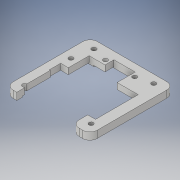
# Autodesk Inventor part: back-cam
Saved by Autodesk Inventor 2019 (Build 230136000, 136)
## iProperties
Created: 2019-02-22
Part Number: back-cam
Material: Generic
Document SubType Name: Modeling
Designer: Tesler
Density: 1 g/cm^3
Appearance: Default
Author: Tesler
Autodesk Inventor part; units mm, degrees
ref_plane "YZ Plane" through (0, 0, 0) normal (1, 0, 0) x (0, 1, 0)
ref_plane "XZ Plane" through (0, 0, 0) normal (0, 1, 0) x (-1, 0, 0)
ref_plane "XY Plane" through (0, 0, 0) normal (0, 0, 1) x (1, 0, 0)
sketch "Sketch1" plane through (0, 0, 0) normal (0, 1, 0) x (-1, 0, 0)
  line L0 (-29.924, 14.3694) -> (-29.924, -45.6306)
  line L1 (29.924, 14.3694) -> (29.924, -45.6306)
  line L2 (-7.574, -27.3788) -> (-7.574, -40.26)
  line L3 (-7.574, -40.26) -> (7.574, -40.26)
  line L4 (29.924, -45.6306) -> (-29.924, -45.6306)
  circle A0 centre (-23.749, 7.365) radius 1.5494
  arc A1 (23.749, 5.8156) -> (23.749, 8.9144) centre (23.749, 7.365) ccw
  circle A2 centre (10.414, -37.085) radius 1.5494
  line L5 (7.574, -33.91) -> (7.574, -40.26)
  circle A3 centre (23.6982, -25.782) radius 1.5494
  line L6 (7.574, -33.91) -> (18.924, -33.91)
  line L7 (-17.105, 14.3694) -> (-17.105, 3.065)
  line L8 (-22.624, 3.065) -> (-17.105, 3.065)
  line L9 (-22.624, 3.065) -> (-22.624, -27.3788)
  line L10 (-7.574, -27.3788) -> (-22.624, -27.3788)
  line L11 (18.924, -19.105) -> (18.924, -33.91)
  line L12 (18.924, -19.105) -> (24.424, -19.105)
  line L13 (23.749, -11.06) -> (24.424, -11.06)
  line L14 (24.424, -19.105) -> (24.424, -11.06)
  line L15 (-29.924, 14.3694) -> (-17.105, 14.3694)
  line L16 (22.1742, 14.3694) -> (29.924, 14.3694)
  line L17 (23.749, 5.8156) -> (23.7568, 5.8156)
  line L18 (23.749, 5.587) -> (23.749, -11.06)
  line L19 (22.1742, 14.3694) -> (22.1742, 8.9144)
  circle A4 centre (-10.414, -37.085) radius 1.5494
  line L20 (23.749, 5.587) -> (23.749, 5.8156)
  line L21 (23.749, 8.9144) -> (22.1742, 8.9144)
  point P0 (0, 0)
  point P1 (0, 0)
  dimension "d0" = 60
  dimension "d7" = 6.2258
  dimension "d8" = 19.8486
  dimension "d9" = 3.0988
  dimension "d12" = 12.8811
  dimension "d14" = 6.175
  dimension "d16" = 12.819
  dimension "d19" = 11
  dimension "d21" = 26.5256
  dimension "d22" = 34.5706
  dimension "d25" = 48.6956
  dimension "d27" = 5.5
  dimension "d28" = 6.175
  dimension "d30" = 7.3
  dimension "d31" = 11.7206
  dimension "d34" = 3.0988
  dimension "d35" = 3.0988
  dimension "d36" = 3.0988
  dimension "d38" = 8.5456
  dimension "d39" = 19.51
  dimension "d40" = 3.0988
  dimension "d41" = 8.5456
  dimension "d42" = 19.51
  dimension "d43" = 52.9956
  dimension "d44" = 6.175
  dimension "d176" = 5.455
  dimension "d177" = 7.7498
  constraints: 44 end point, 13 vertical, 10 horizontal, 5 centre point, 3 perpendicular, 2 point on circle, 1 coincident, 1 parallel, 1 point on line, 1 tangent
  measures "d0" distance of L0.start L0.end
  measures "d7" distance from line of L1 point (23.698, -25.782)
  measures "d8" distance from line of point (23.698, -25.782) L4
  measures "d9" diameter of A3
  measures "d12" distance of L2.start L2.end
  measures "d14" distance from line of A0.centre L0
  measures "d16" distance between parallel lines of L7 L0
  measures "d19" distance between parallel lines of L1 L11
  measures "d21" distance between parallel lines of L4 L12
  measures "d22" distance between parallel lines of L4 L13
  measures "d25" distance between parallel lines of L4 L8
  measures "d27" distance between parallel lines of L14 L1
  measures "d28" distance between parallel lines of L18 L1
  measures "d30" distance between parallel lines of L9 L0
  measures "d31" distance between parallel lines of L4 L6
  measures "d34" diameter of A1
  measures "d35" diameter of A0
  measures "d36" diameter of A2
  measures "d38" distance from line of L4 A2.centre
  measures "d39" distance from line of L1 A2.centre
  measures "d40" diameter of A4
  measures "d41" distance from line of L4 A4.centre
  measures "d42" distance from line of L0 A4.centre
  measures "d43" distance from line of L4 A0.centre
  measures "d44" distance from line of L1 A1.centre
  measures "d176" distance of L16.start L19.end
  measures "d177" distance between parallel lines of L1 L19
extrude "Extrusion1" add sketch "Sketch1" along normal blind 5.08 contours L15 L7 L8 L9 L10 L2 L3 L5 L6 L11 L12 L14 L13 L18 L20 A1 L21 L19 L16 L1 L4 L0 | A0 | A2 | A3 | A4
sketch "Sketch2" plane through (0, 0, 0) normal (0, -1, 0) x (1, 0, 0)
  line L0 (7.574, -40.26) -> (-7.574, -40.26) projected
  line L1 (-29.924, 14.3694) -> (-29.924, -45.6306) projected
  line L2 (-22.1742, 14.3694) -> (-29.924, 14.3694) projected
  line L3 (29.924, 14.3694) -> (17.105, 14.3694) projected
  line L4 (29.924, -45.6306) -> (29.924, 14.3694) projected
  line L5 (-26.924, 10.54) -> (26.924, 10.54)
  line L6 (-26.924, 10.54) -> (-26.924, -40.26)
  line L7 (-26.924, -40.26) -> (26.924, -40.26)
  line L8 (26.924, -40.26) -> (26.924, 10.54)
  point P0 (0, 0)
  dimension "d52" = 53.848
  dimension "d53" = 50.8
  constraints: 8 end point, 2 horizontal, 2 vertical, 1 parallel, 1 perpendicular
  measures "d52" distance of L5.start L5.end
  measures "d53" distance of L7.end L5.end
extrude "Extrusion3" cut sketch "Sketch2" against normal blind 0.7937
extrude "Extrusion2" cut sketch "Sketch1" along normal up to next contours A0 | A2 | A3 | A4
fillet "Fillet1" radius 5.08 4 edges at (29.924, 2.54, 14.3694) (29.924, 2.54, -45.6306) (-29.924, 2.54, -45.6306) (-29.924, 2.54, 14.3694)
fillet "Fillet2" radius 5.08 1 edges at (17.105, 2.54, 14.3694)
sketch "Sketch3" plane through (0, 0.7938, 0) normal (0, -1, 0) x (1, 0, 0)
  line L0 (-26.924, -40.26) -> (-26.924, 10.54) projected
  line L1 (-18.924, -33.91) -> (-7.574, -33.91) projected
  line L2 (-26.924, -40.26) -> (-14.224, -40.26)
  line L3 (-15.7226, -33.91) -> (-26.924, -33.91)
  line L4 (-26.924, -33.91) -> (-26.924, -40.26)
  line L5 (26.924, -40.26) -> (7.574, -40.26) projected
  line L6 (26.924, -40.26) -> (14.224, -40.26)
  line L7 (15.7226, -33.91) -> (26.924, -33.91)
  line L8 (26.924, -33.91) -> (26.924, -40.26)
  line L9 (-14.224, -40.26) -> (-14.224, -35.4086)
  line L10 (14.224, -40.26) -> (14.224, -35.4086)
  line L11 (14.224, -35.4086) -> (15.7226, -33.91)
  line L12 (-14.224, -35.4086) -> (-15.7226, -33.91)
  circle A0 centre (10.414, -37.085) radius 1.5494 projected
  circle A1 centre (-10.414, -37.085) radius 1.5494 projected
  point P0 (0, 0)
  dimension "d58" = 11.2014
  dimension "d59" = 11.2014
  dimension "d60" = 4.8514
  dimension "d61" = 4.8514
  dimension "d64" = 6.35
  dimension "d170" = 3.81
  dimension "d171" = 3.81
  constraints: 20 end point, 3 point on line, 2 horizontal, 2 parallel, 2 vertical, 1 perpendicular
  measures "d58" distance of L3.end L3.start
  measures "d59" distance of L7.start L7.end
  measures "d60" distance of L2.end L9.end
  measures "d61" distance of L6.end L10.end
  measures "d64" distance of L7.end L5.start
  measures "d170" horizontal distance of A1.centre L9.end
  measures "d171" horizontal distance of L10.end A0.centre
extrude "Extrusion4" add sketch "Sketch3" along normal blind 0.7937 contours L0 L3 L1 L12 L9 L2 | L5 L10 L11 L7 L8
sketch "Sketch4" plane through (0, 0, 0) normal (0, -1, 0) x (1, 0, 0)
  line L0 (0, -57.6306) -> (0, 26.3694) projected
  circle A0 centre (-21.3233, -39.7647) radius 1.5875
  line L1 (-15.7226, -33.91) -> (-26.924, -33.91) projected
  line L2 (-14.224, -40.26) -> (-14.224, -35.4086) projected
  circle A1 centre (21.3233, -39.7647) radius 1.5875
  dimension "d172" = 3.175
  dimension "d173" = 5.8547
  dimension "d174" = 7.0993
  constraints: 2 centre point, 1 symmetric about line, 1 other
  measures "d172" diameter of A0
  measures "d173" distance from line of L1 A0.centre
  measures "d174" distance from line of L2 A0.centre
extrude "Extrusion5" cut sketch "Sketch4" against normal up to next
equation "\"d42\" = d39"
body "Solid1"
